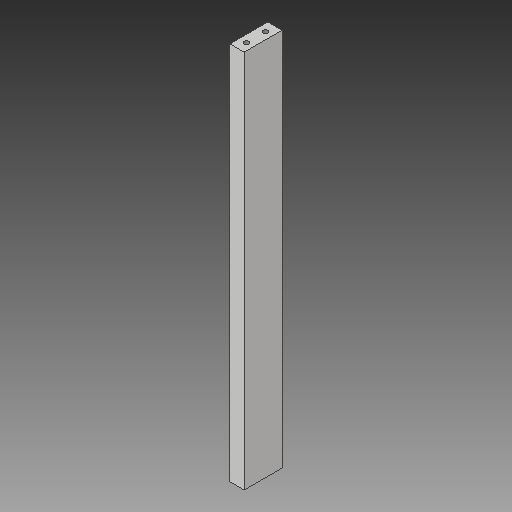
# Autodesk Inventor part: TopPlateRightConnector
Saved by Autodesk Inventor 2019 (Build 230136000, 136)
## iProperties
Created: 2017-12-13
Part Number: TopPlateRightConnector
Material: Generic
Document SubType Name: Modeling
Designer: User
Density: 1 g/cm^3
Appearance: Default
Author: User
Autodesk Inventor part; units mm, degrees
ref_plane "YZ Plane" through (0, 0, 0) normal (1, 0, 0) x (0, 1, 0)
ref_plane "XZ Plane" through (0, 0, 0) normal (0, 1, 0) x (-1, 0, 0)
ref_plane "XY Plane" through (0, 0, 0) normal (0, 0, 1) x (1, 0, 0)
sketch "Sketch1" plane through (0, 0, 0) normal (0, 0, 1) x (1, 0, 0)
  line L0 (0, 0) -> (9.525, 0)
  line L1 (9.525, 0) -> (9.525, 254)
  line L2 (9.525, 254) -> (0, 254)
  line L3 (0, 254) -> (0, 0)
  dimension "d0" = 9.525
  dimension "d1" = 254
  constraints: 8 end point, 2 parallel, 1 horizontal, 1 perpendicular
  measures "d0" distance of L2.end L1.end
  measures "d1" distance of L1.end L0.end
extrude "Extrusion1" add sketch "Sketch1" along normal blind 25.4
sketch "Sketch2" plane through (0, 254, 0) normal (0, 1, 0) x (1, 0, 0)
  line L0 (0, 0) -> (9.525, 0) projected
  line L1 (0, -25.4) -> (9.525, -25.4) projected
  point P0 (4.7625, -19.05)
  point P1 (4.7625, -6.35)
hole "Hole1" at (4.7625, 254, 19.05) at (4.7625, 254, 6.35) direction (0, -1, 0) diameter 3.302 depth 7.62 tip angle 118 thread size "8-32 UNC" class "2B" standard "ANSI Unified Screw Threads"
sketch "Sketch3" plane through (0, 0, 0) normal (0, -1, 0) x (1, 0, 0)
  line L0 (9.525, 0) -> (0, 0) projected
  circle A0 centre (4.7625, 19.05) radius 1.651 projected
  point P0 (4.7625, 6.35)
  constraints: 1 coincident
hole "Hole2" at (4.7625, 0, 19.05) at (4.7625, 0, 6.35) direction (0, 1, 0) diameter 3.302 depth 7.62 tip angle 118 thread size "8-32 UNC" class "2B" standard "ANSI Unified Screw Threads"
body "Solid1"
